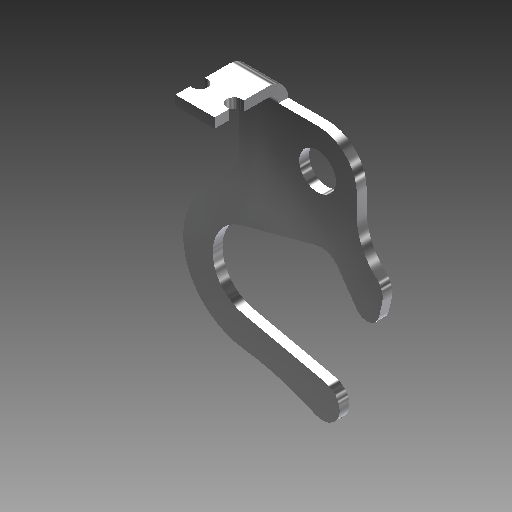
# Autodesk Inventor part: 403-07
Saved by Autodesk Inventor 2019 (Build 230136000, 136)
## iProperties
Company: Autodesk Inc.
Created: 2017-06-27
Part Number: 403-07
Material: Aluminum-6061
Document SubType Name: Sheet Metal
Designer: Autodesk Inc.
Mass: 0.665069 g
Surface Area: 6.25617 cm^2
Volume: 0.246322 cm^3
Density: 2.7 g/cm^3
Flat Pattern Width: 2.03403 cm
Flat Pattern Length: 3.35119 cm
Flat Pattern Area: 6.81642 cm^2
Sheet Metal Rule: Default_mm
Sheet Metal Width: 20.340 mm
Sheet Metal Length: 33.512 mm
Sheet Metal Area: 681.642 mm^2
Appearance: Aluminum - Flat
Author: Inventor
Autodesk Inventor part; units mm, degrees
ref_plane "YZ Plane" through (0, 0, 0) normal (1, 0, 0) x (0, 1, 0)
ref_plane "XZ Plane" through (0, 0, 0) normal (0, 1, 0) x (-1, 0, 0)
ref_plane "XY Plane" through (0, 0, 0) normal (0, 0, 1) x (1, 0, 0)
sketch "Sketch1" plane through (0, 0, 0) normal (0, 0, 1) x (1, 0, 0)
  arc A0 (12.0073, -14.2063) -> (14.25, -13.7671) centre (13.0313, -13.4893) ccw
  arc A1 (10.0296, -11.3818) -> (7.8737, -10.5971) centre (8.3913, -12.529) ccw
  arc A2 (0.2652, -12.6358) -> (0.4372, -20.4052) centre (1.3005, -16.4995) ccw
  circle A3 centre (8.5, -24) radius 1.75
  arc A4 (8.931, -22.3039) -> (7.6516, -22) centre (-1.4138, -63.01) ccw
  arc A5 (-0.5845, -7.856) -> (0, -6.25) centre (-2.4984, -6.25) ccw
  line L0 (0, 0) -> (-8.9372, 0) construction
  arc A6 (12, -4) -> (8, 0) centre (8, -4) ccw
  arc A7 (12, -6) -> (14.0314, -10.5) centre (18, -6) ccw
  arc A8 (-4.0618, -12) -> (0.3968, -23.4409) centre (1.3005, -16.4995) ccw
  line L1 (0, 0) -> (0, -6.25)
  line L2 (-0.5845, -7.856) -> (-4.0618, -12)
  line L3 (8, 0) -> (0, 0)
  line L4 (12, -4) -> (12, -6)
  line L5 (12.0073, -14.2063) -> (10.0296, -11.3818)
  line L6 (14.25, -13.7671) -> (14.5958, -12.25)
  arc A9 (14.5958, -12.25) -> (14.0314, -10.5) centre (12.8408, -11.85) ccw
  line L7 (0.2652, -12.6358) -> (7.8737, -10.5971)
  line L8 (7.6516, -22) -> (0.4372, -20.4052)
  arc A10 (7.7587, -25.5853) -> (0.3968, -23.4409) centre (-2.8308, -48.2317) ccw
  point P0 (7.0822, -25.0258)
  point P1 (8.931, -22.3039)
  dimension "d74" = 6.25
  dimension "d76" = 8
  dimension "d77" = 4
  dimension "d78" = 4
  dimension "d79" = 2
  dimension "d80" = 6
  dimension "d81" = 1.8
  dimension "d82" = 1.25
  dimension "d83" = 2
  dimension "d84" = 4
  dimension "d85" = 2.4984
  dimension "d86" = 7
  dimension "d87" = 140
  dimension "d88" = 12
  dimension "d89" = 10.5
  dimension "d90" = 1.75
  dimension "d91" = 14.25
  dimension "d93" = 15
  dimension "d94" = 55
  dimension "d95" = 24
  dimension "d96" = 8.5
  dimension "d97" = 3.5
  dimension "d98" = 25
  dimension "d102" = 22
  dimension "d104" = 42
  measures "d74" distance of L1.start L1.end
  measures "d76" distance of L3.start L1.start
  measures "d77" radius of A6
  measures "d78" distance from line of L3 L4.start
  measures "d79" distance of L4.start L4.end
  measures "d80" radius of A7
  measures "d81" radius of A9
  measures "d82" radius of A0
  measures "d83" radius of A1
  measures "d84" radius of A2
  measures "d85" radius of A5
  measures "d86" radius of A8
  measures "d87" angle of L1 L2
  measures "d88" vertical distance of L0.start L2.end
  measures "d89" vertical distance of L3.start A7.end
  measures "d90" vertical distance of A7.end L6.end
  measures "d91" distance from line of L1 L6.start
  measures "d93" angle of L7 L3
  measures "d94" angle of L3 L5
  measures "d95" distance from line of L3 A3.centre
  measures "d96" horizontal distance of L0.start A3.centre
  measures "d97" diameter of A3
  measures "d98" radius of A10
  measures "d102" distance from line of L3 L8.start
  measures "d104" radius of A4
extrude "Plate1" add sketch "Sketch1" against normal blind 1
ref_plane "Work Plane1" through (0, 1, 0) normal (0, 1, 0) x (1, 0, 0)
sketch "Sketch2" plane through (0, 1, 0) normal (0, 1, 0) x (-1, 0, 0)
  line L0 (0, 0) -> (-4, 0)
  line L1 (-4, 0) -> (-4, 6.5)
  line L2 (-4, 6.5) -> (0, 6.5)
  line L3 (0, 6.5) -> (0, 0)
  line L4 (0, 5) -> (-0.25, 5)
  arc A0 (-0.25, 5) -> (-0.25, 3.5) centre (-0.25, 4.25) ccw
  line L5 (-0.25, 3.5) -> (0, 3.5)
  line L6 (-4, 5) -> (-3.75, 5)
  arc A1 (-3.75, 3.5) -> (-3.75, 5) centre (-3.75, 4.25) ccw
  line L7 (-3.75, 3.5) -> (-4, 3.5)
  dimension "d52" = 4
  dimension "d53" = 6.5
  dimension "d55" = 3.5
  dimension "d56" = 4.25
  dimension "d57" = 0.75
  measures "d52" distance of L1.end L2.end
  measures "d53" distance of L0.end L1.end
  measures "d55" distance of A1.centre A0.centre
  measures "d56" distance from line of L0 A1.centre
  measures "d57" radius of A1
sheet face with bend "Face2" sketch "Sketch2" thickness 1 toward (0, 1, 0) bend radius 1 relief round relief width 1 relief depth 0.5 contours L0 L1 L7 A1 L6 L2 L3 L4 A0 L5
bend "Bend1"
hole "Hole1" at (8, -4, 0) direction (0, 0, -1) diameter 3.75 end through all
equation "\"d70\" = Thickness"
equation "\"d72\" = Thickness"
equation "\"d58\" = BendRadius"
equation "\"d61\" = MinimumRemnant"
equation "\"d59\" = BendReliefWidth"
equation "\"d60\" = BendReliefDepth"
equation "\"d62\" = BendRadius"
equation "\"BendRadius\" = Thickness"
equation "\"BendReliefWidth\" = Thickness"
equation "\"BendReliefDepth\" = 0.5 * Thickness"
equation "\"CornerReliefSize\" = 4 * Thickness"
equation "\"MinimumRemnant\" = 2 * Thickness"
equation "\"TransitionRadius\" = BendRadius"
equation "\"JacobiRadiusSize\" = BendRadius"
equation "\"GapSize\" = Thickness"
equation "\"d51\" = BendRadius"
equation "\"Thickness\" = 1"
body "Solid1"
